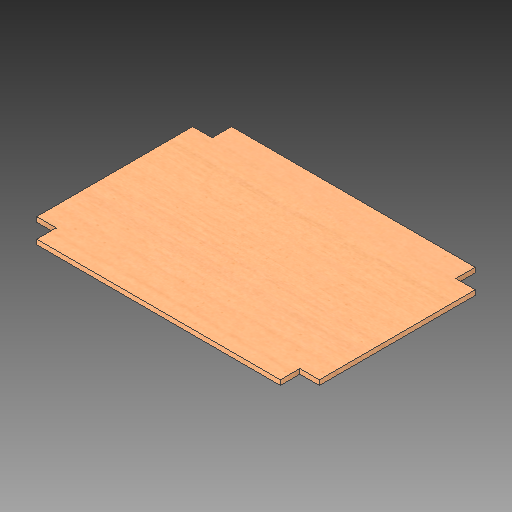
# Autodesk Inventor part: etage-carte
Saved by Autodesk Inventor 2019 (Build 230136000, 136)
## iProperties
Created: 2018-04-06
Part Number: etage-carte
Material: Générique
Document SubType Name: Modeling
Designer: franc
Density: 1 g/cm^3
Appearance: Par défaut
Author: franc
Autodesk Inventor part; units mm, degrees
ref_plane "YZ Plane" through (0, 0, 0) normal (1, 0, 0) x (0, 1, 0)
ref_plane "XZ Plane" through (0, 0, 0) normal (0, 1, 0) x (-1, 0, 0)
ref_plane "XY Plane" through (0, 0, 0) normal (0, 0, 1) x (1, 0, 0)
sketch "Sketch1" plane through (0, 0, 0) normal (0, 1, 0) x (-1, 0, 0)
  line L0 (119.8469, 90.3599) -> (-117.1337, 90.3599)
  line L1 (-117.1337, 90.3599) -> (-117.1337, 70.3599)
  line L2 (-117.1337, 70.3599) -> (-137.1337, 70.3599)
  line L3 (-137.1337, 70.3599) -> (-137.1337, -89.6401)
  line L4 (-137.1337, -89.6401) -> (-117.1337, -89.6401)
  line L5 (-117.1337, -89.6401) -> (-117.1337, -109.6401)
  line L6 (-117.1337, -109.6401) -> (132.8663, -109.6401)
  line L7 (132.8663, -109.6401) -> (132.8663, -89.6401)
  line L8 (132.8663, -89.6401) -> (152.8663, -89.6401)
  line L9 (152.8663, -89.6401) -> (152.8663, 70.3599)
  line L10 (152.8663, 70.3599) -> (132.8663, 70.3599)
  line L11 (132.8663, 90.3599) -> (117.0353, 90.3599)
  line L12 (132.8663, 70.3599) -> (132.8663, 90.3599)
  dimension "d13" = 290
  dimension "d14" = 200
  dimension "d15" = 20
  dimension "d16" = 20
  dimension "d17" = 20
  dimension "d18" = 20
  constraints: 26 end point, 10 point on line, 7 perpendicular, 1 horizontal, 1 vertical
  measures "d13" distance between parallel lines of L3 L9
  measures "d14" distance between parallel lines of L6 L0
  measures "d15" distance of L0.end L1.end
  measures "d16" distance of L1.end L2.end
  measures "d17" distance of L4.end L5.end
  measures "d18" distance of L7.end L8.end
extrude "Extrusion1" add sketch "Sketch1" along normal blind 5
body "Solid1"
